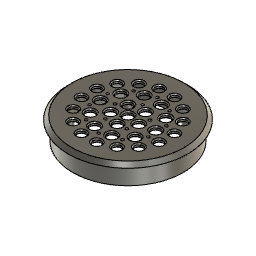
Griglietta aria tonda 60mm v3 (Autodesk Fusion 360 design; units mm, degrees)
Autodesk Fusion 360 part; units mm, degrees
cylinder "PrimitivaCilindro1" add diameter 70 height 2 placed x (1, 0, 0) y (0, 1, 0) z (0, 0, 1) at (0, 0, 0)
sketch "Schizzo2" plane through (0, 0, 2) normal (0, 0, 1) x (-1, 0, 0)
  circle A0 centre (0, 0) radius 35
  circle A1 centre (5, -5) radius 2.4718
  circle A2 centre (6.3004, 3.2102) radius 2.4718
  circle A3 centre (-1.1062, 6.984) radius 2.4718
  circle A4 centre (-6.984, 1.1062) radius 2.4718
  circle A5 centre (-3.2102, -6.3004) radius 2.4718
  circle A6 centre (12.1495, -8.2504) radius 2.5
  circle A7 centre (14.6786, 0.4666) radius 2.5
  circle A8 centre (11.601, 9.0053) radius 2.5
  circle A9 centre (4.0922, 14.1043) radius 2.5
  circle A10 centre (-4.9797, 13.816) radius 2.5
  circle A11 centre (-12.1495, 8.2504) radius 2.5
  circle A12 centre (-14.6786, -0.4666) radius 2.5
  circle A13 centre (-11.601, -9.0053) radius 2.5
  circle A14 centre (-4.0922, -14.1043) radius 2.5
  circle A15 centre (4.9797, -13.816) radius 2.5
  line L0 (16, -16) -> (-16, 16) construction
  circle A16 centre (21.1596, 4.1773) radius 2.2588
  circle A17 centre (17.9503, 11.9568) radius 2.2588
  circle A18 centre (12.0083, 17.9159) radius 2.2588
  circle A19 centre (4.2381, 21.1475) radius 2.2588
  circle A20 centre (-4.1773, 21.1596) radius 2.2588
  circle A21 centre (-11.9568, 17.9503) radius 2.2588
  circle A22 centre (-17.9159, 12.0083) radius 2.2588
  circle A23 centre (-21.1475, 4.2381) radius 2.2588
  circle A24 centre (-21.1596, -4.1773) radius 2.2588
  circle A25 centre (-17.9503, -11.9568) radius 2.2588
  circle A26 centre (-12.0083, -17.9159) radius 2.2588
  circle A27 centre (-4.2381, -21.1475) radius 2.2588
  circle A28 centre (4.1773, -21.1596) radius 2.2588
  circle A29 centre (11.9568, -17.9503) radius 2.2588
  circle A30 centre (17.9159, -12.0083) radius 2.2588
  circle A31 centre (21.1475, -4.2381) radius 2.2588
  dimension "d4" = 360
  dimension "d5" = 5
  dimension "d7" = 360
  constraint coincident L0 A0.centre
  constraint coincident A0.centre origin
  measures "d5" diameter of A6
extrude "Estrusione4" cut sketch "Schizzo2" against normal blind 10 contours A1 | A2 | A3 | A4 | A5 | A6 | A7 | A8 | A9 | A10 | A11 | A12 | A13 | A14 | A15 | A16 | A17 | A18 | A19 | A20 | A21 | A22 | A23 | A24 | A25 | A26 | A27 | A28 | A29 | A30 | A31
sketch "Schizzo3" plane through (0, 0, 0) normal (0, 0, -1) x (1, 0, 0)
  circle A0 centre (0, 0) radius 35
  circle A1 centre (0, 0) radius 30.1
  circle A2 centre (0, 0) radius 29.4
  circle A3 centre (-12.0083, 17.9159) radius 2.2588
  circle A4 centre (3.2102, -6.3004) radius 2.4718
  circle A5 centre (-14.6786, 0.4666) radius 2.5
  circle A6 centre (21.1596, -4.1773) radius 2.2588
  circle A7 centre (21.1475, 4.2381) radius 2.2588
  circle A8 centre (4.9797, 13.816) radius 2.5
  circle A9 centre (11.601, -9.0053) radius 2.5
  circle A10 centre (-21.1475, -4.2381) radius 2.2588
  circle A11 centre (-4.1773, -21.1596) radius 2.2588
  circle A12 centre (14.6786, -0.4666) radius 2.5
  circle A13 centre (-17.9503, 11.9568) radius 2.2588
  circle A14 centre (11.9568, 17.9503) radius 2.2588
  circle A15 centre (1.1062, 6.984) radius 2.4718
  circle A16 centre (-6.3004, 3.2102) radius 2.4718
  circle A17 centre (4.2381, -21.1475) radius 2.2588
  circle A18 centre (4.1773, 21.1596) radius 2.2588
  circle A19 centre (-11.601, 9.0053) radius 2.5
  circle A20 centre (-4.0922, 14.1043) radius 2.5
  circle A21 centre (17.9503, -11.9568) radius 2.2588
  circle A22 centre (17.9159, 12.0083) radius 2.2588
  circle A23 centre (12.1495, 8.2504) radius 2.5
  circle A24 centre (-4.9797, -13.816) radius 2.5
  circle A25 centre (-17.9159, -12.0083) radius 2.2588
  circle A26 centre (-11.9568, -17.9503) radius 2.2588
  circle A27 centre (4.0922, -14.1043) radius 2.5
  circle A28 centre (-21.1596, 4.1773) radius 2.2588
  circle A29 centre (12.0083, -17.9159) radius 2.2588
  circle A30 centre (6.984, 1.1062) radius 2.4718
  circle A31 centre (-5, -5) radius 2.4718
  circle A32 centre (-12.1495, -8.2504) radius 2.5
  circle A33 centre (-4.2381, 21.1475) radius 2.2588
  dimension "d17" = 60.2
  dimension "d18" = 58.8
  constraint concentric A0 A1
  constraint concentric A1 A2
  measures "d17" diameter of A1
  measures "d18" diameter of A2
extrude "Estrusione2" add sketch "Schizzo3" along normal blind 10 contours A1
fillet "Raccordo2" radius 1 1 edges at (-32.6315, -12.6565, 2)
sketch "Schizzo5" plane through (0, 0, 0) normal (0, 0, 1) x (1, 0, 0)
  line L0 (20, 20) -> (-20, 20)
  line L1 (-20, 20) -> (-20, -20)
  line L2 (20, -20) -> (20, 20)
  line L3 (20, 20) -> (-20, -20) construction
  line L4 (-20, 20) -> (20, -20) construction
  line L5 (18.5, 18.5) -> (-18.5, 18.5)
  line L6 (-18.5, 18.5) -> (-18.5, -18.5)
  line L7 (-18.5, -18.5) -> (18.5, -18.5)
  line L8 (18.5, -18.5) -> (18.5, 18.5)
  line L9 (18.5, 18.5) -> (-18.5, -18.5) construction
  line L10 (-18.5, 18.5) -> (18.5, -18.5) construction
  line L11 (16, 16) -> (-16, 16)
  line L12 (-16, 16) -> (-16, -16)
  line L13 (-16, -16) -> (16, -16)
  line L14 (16, -16) -> (16, 16)
  line L15 (16, 16) -> (-16, -16) construction
  line L16 (-16, 16) -> (16, -16) construction
  circle A0 centre (-20, -20) radius 2
  circle A1 centre (-18.5, -18.5) radius 2
  circle A2 centre (-16, -16) radius 2
  circle A3 centre (0, 0) radius 29.4
  circle A4 centre (20, -20) radius 2
  circle A5 centre (20, -20) radius 2
  circle A6 centre (18.5, -18.5) radius 2
  circle A7 centre (16, -16) radius 2
  circle A8 centre (-20, 20) radius 2
  circle A9 centre (-18.5, 18.5) radius 2
  circle A10 centre (-16, 16) radius 2
  circle A11 centre (16, 16) radius 2
  circle A12 centre (18.5, 18.5) radius 2
  circle A13 centre (20, 20) radius 2
  circle A14 centre (-16, 16) radius 0.5
  circle A15 centre (-18.5, 18.5) radius 0.5
  circle A16 centre (-20, 20) radius 0.5
  circle A17 centre (16, 16) radius 0.5
  circle A18 centre (18.5, 18.5) radius 0.5
  circle A19 centre (20, 20) radius 0.5
  circle A20 centre (-20, -20) radius 0.5
  circle A21 centre (-18.5, -18.5) radius 0.5
  circle A22 centre (-16, -16) radius 0.5
  circle A23 centre (16, -16) radius 0.5
  circle A24 centre (18.5, -18.5) radius 0.5
  circle A25 centre (20, -20) radius 0.5
  dimension "d27" = 40
  dimension "d28" = 40
  dimension "d29" = 37
  dimension "d30" = 37
  dimension "d31" = 32
  dimension "d32" = 32
  dimension "d41" = 4
  dimension "d42" = 4
  dimension "d43" = 4
  dimension "d44" = 58.8
  dimension "d45" = 4
  dimension "d46" = 4
  dimension "d47" = 4
  dimension "d48" = 4
  dimension "d49" = 4
  dimension "d50" = 4
  dimension "d51" = 4
  dimension "d52" = 4
  dimension "d53" = 4
  dimension "d54" = 4
  dimension "d55" = 1
  dimension "d56" = 1
  dimension "d57" = 1
  dimension "d58" = 1
  dimension "d59" = 1
  dimension "d60" = 1
  dimension "d61" = 1
  dimension "d62" = 1
  dimension "d63" = 1
  dimension "d64" = 1
  dimension "d65" = 1
  dimension "d66" = 1
  constraint horizontal L0
  constraint perpendicular L0 L1
  constraint parallel L1 L2
  constraint coincident L3 A3.centre
  constraint coincident L4 A3.centre
  constraint coincident A3.centre origin
  constraint horizontal L5
  constraint perpendicular L5 L6
  constraint parallel L5 L7
  constraint parallel L6 L8
  constraint coincident L9 A3.centre
  constraint coincident L10 A3.centre
  constraint horizontal L11
  constraint perpendicular L11 L12
  constraint parallel L11 L13
  constraint parallel L12 L14
  constraint coincident L15 A3.centre
  constraint coincident L16 A3.centre
  constraint coincident L1.end L3.end
  constraint coincident L6.end L7.start
  constraint coincident L12.end L13.start
  constraint coincident L2.start L4.end
  constraint coincident L7.end L8.start
  constraint coincident L13.end L14.start
  constraint coincident L0.end L1.start
  constraint coincident L5.end L6.start
  constraint coincident L11.end L12.start
  constraint coincident L11.start L14.end
  constraint coincident L5.start L8.end
  constraint coincident L0.start L2.end
  constraint concentric A10 A14
  constraint concentric A9 A15
  constraint concentric A8 A16
  constraint concentric A11 A17
  constraint concentric A12 A18
  constraint concentric A13 A19
  constraint concentric A0 A20
  constraint concentric A1 A21
  constraint concentric A2 A22
  constraint concentric A7 A23
  constraint concentric A6 A24
  constraint concentric A5 A25
  measures "d27" distance of L1.end L2.start
  measures "d28" distance of L0.end L1.end
  measures "d29" distance of L6.end L7.end
  measures "d30" distance of L5.end L6.end
  measures "d31" distance of L12.end L13.end
  measures "d32" distance of L11.end L12.end
  measures "d41" diameter of A0
  measures "d42" diameter of A1
  measures "d43" diameter of A2
  measures "d44" diameter of A3
  measures "d45" diameter of A4
  measures "d46" diameter of A5
  measures "d47" diameter of A6
  measures "d48" diameter of A7
  measures "d49" diameter of A8
  measures "d50" diameter of A9
  measures "d51" diameter of A10
  measures "d52" diameter of A11
  measures "d53" diameter of A12
  measures "d54" diameter of A13
  measures "d55" diameter of A14
  measures "d56" diameter of A15
  measures "d57" diameter of A16
  measures "d58" diameter of A17
  measures "d59" diameter of A18
  measures "d60" diameter of A19
  measures "d61" diameter of A20
  measures "d62" diameter of A21
  measures "d63" diameter of A22
  measures "d64" diameter of A23
  measures "d65" diameter of A24
  measures "d66" diameter of A25
extrude "Estrusione5" add sketch "Schizzo5" against normal blind 10 contours L0 L1 A8 A15 A16 | L0 A8 A9 | L0 A8 A9 A16 | L0 L5 A8 A9 A15 | A3 A8 A9 A16 | L1 A8 A9 A16 | L0 A12 A13 | L0 L5 A12 A13 A18 | L5 L6 A9 A10 A15 | L1 L6 A8 A9 A15 | L1 A8 A9 | L0 A12 A13 A19 | L0 L2 A13 A18 A19 | A3 A12 A13 A19 | L5 L8 A11 A12 A18 | L11 L12 A9 A10 A14 | A9 A10 | L11 L14 A11 A12 A17 | A11 A12 | L11 L12 A10 A14 | A0 A1 A3 A20 | L1 L6 A0 A1 A21 | L1 A0 A1 | L2 A12 A13 A19 | L2 L8 A12 A13 A18 | L11 L14 A11 A17 | L2 A12 A13 | L1 A0 A1 A20 | L6 L7 A1 A2 A21 | L1 A0 A1 A20 A21 | L12 L13 A2 A22 | L12 L13 A1 A2 A22 | A3 A4 A5 A6 A25 | L7 A0 A1 A21 | A1 A2 | L2 L8 A4 A5 A6 A24 | L7 L8 A6 A7 A24 | L13 L14 A6 A7 A23 | L13 L14 A7 A23 | L2 A4 A5 A6 A25 | L2 A4 A5 A6 | L7 A4 A5 A6 A24 | L2 A4 A5 A6 A24 A25 | A6 A7
extrude "Estrusione6" add sketch "Schizzo5" against normal blind 5 contours L7 L8 A4 A5 A24 | L7 L8 A24 | L13 L14 A23 | L13 L14 A23 | A4 A5 A24 | L2 A6 A25 | A6 A25 | L2 A6 A25
extrude "Estrusione7" add 3 faces at (-18.3961, -18.32, 0) (-19.8961, -19.82, 0) (-15.9875, -16.1588, 0) along direction (0, 0, -1) blind 5
extrude "Estrusione8" add 3 faces at (-15.8463, 15.9752, 0) (-18.3961, 18.68, 0) (-19.8961, 20.18, 0) along direction (0, 0, -1) blind 5
extrude "Estrusione9" add 3 faces at (16.1368, 15.8392, 0) (18.6039, 18.68, 0) (20.1039, 20.18, 0) along direction (0, 0, -1) blind 5
sketch "Schizzo6" plane through (0, 0, 0) normal (0, 0, -1) x (1, 0, 0)
  circle A0 centre (-12.0083, 17.9159) radius 2.2588
  circle A1 centre (3.2102, -6.3004) radius 2.4718
  circle A2 centre (-14.6786, 0.4666) radius 2.5
  circle A3 centre (21.1596, -4.1773) radius 2.2588
  circle A4 centre (21.1475, 4.2381) radius 2.2588
  circle A5 centre (4.9797, 13.816) radius 2.5
  circle A6 centre (11.601, -9.0053) radius 2.5
  circle A7 centre (-21.1475, -4.2381) radius 2.2588
  circle A8 centre (-4.1773, -21.1596) radius 2.2588
  circle A9 centre (14.6786, -0.4666) radius 2.5
  circle A10 centre (-17.9503, 11.9568) radius 2.2588
  circle A11 centre (11.9568, 17.9503) radius 2.2588
  circle A12 centre (1.1062, 6.984) radius 2.4718
  circle A13 centre (-6.3004, 3.2102) radius 2.4718
  circle A14 centre (4.2381, -21.1475) radius 2.2588
  circle A15 centre (4.1773, 21.1596) radius 2.2588
  circle A16 centre (-11.601, 9.0053) radius 2.5
  circle A17 centre (-4.0922, 14.1043) radius 2.5
  circle A18 centre (17.9503, -11.9568) radius 2.2588
  circle A19 centre (17.9159, 12.0083) radius 2.2588
  circle A20 centre (12.1495, 8.2504) radius 2.5
  circle A21 centre (-4.9797, -13.816) radius 2.5
  circle A22 centre (-17.9159, -12.0083) radius 2.2588
  circle A23 centre (-11.9568, -17.9503) radius 2.2588
  circle A24 centre (4.0922, -14.1043) radius 2.5
  circle A25 centre (-21.1596, 4.1773) radius 2.2588
  circle A26 centre (12.0083, -17.9159) radius 2.2588
  circle A27 centre (6.984, 1.1062) radius 2.4718
  circle A28 centre (-5, -5) radius 2.4718
  circle A29 centre (-12.1495, -8.2504) radius 2.5
  circle A30 centre (-4.2381, 21.1475) radius 2.2588
  arc A31 (20.449, 18.051) -> (21.9506, 19.5584) centre (20, 20) ccw
  arc A32 (17.9114, 16.5886) -> (20.449, 18.051) centre (18.5, 18.5) ccw
  arc A33 (16.5886, 17.9114) -> (17.9114, 16.5886) centre (16, 16) ccw
  arc A34 (18.051, 20.449) -> (16.5886, 17.9114) centre (18.5, 18.5) ccw
  arc A35 (19.5584, 21.9506) -> (18.051, 20.449) centre (20, 20) ccw
  arc A36 (19.5584, 21.9506) -> (-19.5584, 21.9506) centre (0, 0) ccw
  arc A37 (-18.051, 20.449) -> (-19.5584, 21.9506) centre (-20, 20) ccw
  arc A38 (-16.5886, 17.9114) -> (-18.051, 20.449) centre (-18.5, 18.5) ccw
  arc A39 (-17.9114, 16.5886) -> (-16.5886, 17.9114) centre (-16, 16) ccw
  arc A40 (-20.449, 18.051) -> (-17.9114, 16.5886) centre (-18.5, 18.5) ccw
  arc A41 (-21.9506, 19.5584) -> (-20.449, 18.051) centre (-20, 20) ccw
  arc A42 (-21.9506, 19.5584) -> (-21.9506, -19.5584) centre (0, 0) ccw
  arc A43 (-20.449, -18.051) -> (-21.9506, -19.5584) centre (-20, -20) ccw
  arc A44 (-17.9114, -16.5886) -> (-20.449, -18.051) centre (-18.5, -18.5) ccw
  arc A45 (-16.5886, -17.9114) -> (-17.9114, -16.5886) centre (-16, -16) ccw
  arc A46 (-18.051, -20.449) -> (-16.5886, -17.9114) centre (-18.5, -18.5) ccw
  arc A47 (-19.5584, -21.9506) -> (-18.051, -20.449) centre (-20, -20) ccw
  arc A48 (-19.5584, -21.9506) -> (19.5584, -21.9506) centre (0, 0) ccw
  arc A49 (18.051, -20.449) -> (19.5584, -21.9506) centre (20, -20) ccw
  arc A50 (16.5886, -17.9114) -> (18.051, -20.449) centre (18.5, -18.5) ccw
  arc A51 (17.9114, -16.5886) -> (16.5886, -17.9114) centre (16, -16) ccw
  arc A52 (20.449, -18.051) -> (17.9114, -16.5886) centre (18.5, -18.5) ccw
  arc A53 (21.9506, -19.5584) -> (20.449, -18.051) centre (20, -20) ccw
  arc A54 (21.9506, -19.5584) -> (21.9506, 19.5584) centre (0, 0) ccw
  arc A55 (20, -20) -> (20, 20) centre (-17.5, 0) ccw
  arc A56 (-20, -20) -> (20, -20) centre (0, 17.5134) ccw
  arc A57 (-20, 20) -> (-20, -20) centre (21.0472, 0) ccw
  arc A58 (20, 20) -> (-20, 20) centre (0, -17.5) ccw
  arc A59 (20.2824, 20.5294) -> (-20.2824, 20.5294) centre (0, -17.5) ccw
  arc A60 (-20.4538, -20.4375) -> (20.4432, -20.4432) centre (0, 17.5134) ccw
  arc A61 (20.4432, -20.4432) -> (20.4432, 20.4432) centre (-17.5, 0) ccw
  arc A62 (20.4432, 20.4432) -> (-20.4538, 20.4375) centre (0, -17.5) ccw
  arc A63 (-20.4538, 20.4375) -> (-20.4538, -20.4375) centre (21.0472, 0) ccw
  dimension "d77" = 0.6
  dimension "d78" = 0.6
  constraint coincident A49.centre A53.centre
  constraint coincident A31.centre A35.centre
  constraint coincident A43.centre A47.centre
  constraint tangent A40 A57
  constraint coincident A37.centre A41.centre
extrude "Estrusione10" add sketch "Schizzo6" along normal blind 9.4 contours A31 A53 A55 A61 | A35 A37 A58 A59 A62 | A47 A49 A56 A60 | A41 A43 A57 A63
sketch "Schizzo7" plane through (0, 0, 0) normal (0, 0, -1) x (1, 0, 0)
  circle A0 centre (-12.0083, 17.9159) radius 2.2588
  circle A1 centre (3.2102, -6.3004) radius 2.4718
  circle A2 centre (-14.6786, 0.4666) radius 2.5
  circle A3 centre (21.1596, -4.1773) radius 2.2588
  circle A4 centre (21.1475, 4.2381) radius 2.2588
  circle A5 centre (4.9797, 13.816) radius 2.5
  circle A6 centre (11.601, -9.0053) radius 2.5
  circle A7 centre (-21.1475, -4.2381) radius 2.2588
  circle A8 centre (-4.1773, -21.1596) radius 2.2588
  circle A9 centre (14.6786, -0.4666) radius 2.5
  circle A10 centre (-17.9503, 11.9568) radius 2.2588
  circle A11 centre (11.9568, 17.9503) radius 2.2588
  circle A12 centre (1.1062, 6.984) radius 2.4718
  circle A13 centre (-6.3004, 3.2102) radius 2.4718
  circle A14 centre (4.2381, -21.1475) radius 2.2588
  circle A15 centre (4.1773, 21.1596) radius 2.2588
  circle A16 centre (-11.601, 9.0053) radius 2.5
  circle A17 centre (-4.0922, 14.1043) radius 2.5
  circle A18 centre (17.9503, -11.9568) radius 2.2588
  circle A19 centre (17.9159, 12.0083) radius 2.2588
  circle A20 centre (12.1495, 8.2504) radius 2.5
  circle A21 centre (-4.9797, -13.816) radius 2.5
  circle A22 centre (-17.9159, -12.0083) radius 2.2588
  circle A23 centre (-11.9568, -17.9503) radius 2.2588
  circle A24 centre (4.0922, -14.1043) radius 2.5
  circle A25 centre (-21.1596, 4.1773) radius 2.2588
  circle A26 centre (12.0083, -17.9159) radius 2.2588
  circle A27 centre (6.984, 1.1062) radius 2.4718
  circle A28 centre (-5, -5) radius 2.4718
  circle A29 centre (-12.1495, -8.2504) radius 2.5
  circle A30 centre (-4.2381, 21.1475) radius 2.2588
  arc A31 (-20.8364, 18.1833) -> (-20.8364, -18.1833) centre (21.0472, 0) ccw
  arc A32 (-20.449, -18.051) -> (-20.8364, -18.1833) centre (-20, -20) ccw
  arc A33 (-17.9114, -16.5886) -> (-20.449, -18.051) centre (-18.5, -18.5) ccw
  arc A34 (-16.5886, -17.9114) -> (-17.9114, -16.5886) centre (-16, -16) ccw
  arc A35 (-18.051, -20.449) -> (-16.5886, -17.9114) centre (-18.5, -18.5) ccw
  arc A36 (-18.2135, -20.8991) -> (-18.051, -20.449) centre (-20, -20) ccw
  arc A37 (-18.2135, -20.8991) -> (18.2135, -20.8991) centre (0, 17.5134) ccw
  arc A38 (18.051, -20.449) -> (18.2135, -20.8991) centre (20, -20) ccw
  arc A39 (16.5886, -17.9114) -> (18.051, -20.449) centre (18.5, -18.5) ccw
  arc A40 (17.9114, -16.5886) -> (16.5886, -17.9114) centre (16, -16) ccw
  arc A41 (20.449, -18.051) -> (17.9114, -16.5886) centre (18.5, -18.5) ccw
  arc A42 (20.8994, -18.2136) -> (20.449, -18.051) centre (20, -20) ccw
  arc A43 (20.8994, -18.2136) -> (20.8994, 18.2136) centre (-17.5, 0) ccw
  arc A44 (20.449, 18.051) -> (20.8994, 18.2136) centre (20, 20) ccw
  arc A45 (17.9114, 16.5886) -> (20.449, 18.051) centre (18.5, 18.5) ccw
  arc A46 (16.5886, 17.9114) -> (17.9114, 16.5886) centre (16, 16) ccw
  arc A47 (18.051, 20.449) -> (16.5886, 17.9114) centre (18.5, 18.5) ccw
  arc A48 (18.2136, 20.8994) -> (18.051, 20.449) centre (20, 20) ccw
  arc A49 (18.2136, 20.8994) -> (-18.2136, 20.8994) centre (0, -17.5) ccw
  arc A50 (-18.051, 20.449) -> (-18.2136, 20.8994) centre (-20, 20) ccw
  arc A51 (-16.5886, 17.9114) -> (-18.051, 20.449) centre (-18.5, 18.5) ccw
  arc A52 (-17.9114, 16.5886) -> (-16.5886, 17.9114) centre (-16, 16) ccw
  arc A53 (-20.449, 18.051) -> (-17.9114, 16.5886) centre (-18.5, 18.5) ccw
  arc A54 (-20.8364, 18.1833) -> (-20.449, 18.051) centre (-20, 20) ccw
  circle A55 centre (0, 0) radius 2.5
  circle A56 centre (-10, -13) radius 0.75
  circle A57 centre (-0.449, -16.3951) radius 0.75
  circle A58 centre (9.2736, -13.5278) radius 0.75
  circle A59 centre (15.4539, -5.4933) radius 0.75
  circle A60 centre (15.7314, 4.6394) radius 0.75
  circle A61 centre (10, 13) radius 0.75
  circle A62 centre (0.449, 16.3951) radius 0.75
  circle A63 centre (-9.2736, 13.5278) radius 0.75
  circle A64 centre (-15.4539, 5.4933) radius 0.75
  circle A65 centre (-15.7314, -4.6394) radius 0.75
  circle A66 centre (-1, -9) radius 0.75
  circle A67 centre (8.2505, -3.7322) radius 0.75
  circle A68 centre (6.0991, 6.6934) radius 0.75
  circle A69 centre (-4.4811, 7.8689) radius 0.75
  circle A70 centre (-8.8685, -1.8301) radius 0.75
  dimension "d81" = 5
  dimension "d82" = 1.5
  dimension "d84" = 360
  dimension "d85" = 1.5
  dimension "d87" = 360
  constraint coincident A55.centre origin
  measures "d81" diameter of A55
  measures "d82" diameter of A56
  measures "d85" diameter of A66
extrude "Estrusione11" cut sketch "Schizzo7" against normal blind 4 contours A55 | A56 | A57 | A58 | A59 | A60 | A61 | A62 | A63 | A64 | A65 | A66 | A67 | A68 | A69 | A70
sketch "Schizzo8" plane through (0, 0, 0) normal (0, 0, 1) x (1, 0, 0)
  circle A0 centre (0, 0) radius 28.25
  dimension "d90" = 56.5
  constraint coincident A0.centre origin
  measures "d90" diameter of A0
split_face "DividiFaccia1" 4 faces at (26.605, 3.5465, 0) (-26.3601, 3.5319, 0) (3.5465, 26.604, 0) (3.5465, -26.605, 0) by curves path "Schizzo8" along A0
extrude "Estrusione12" add 4 faces at (-23.2271, -16.6422, 0) (-16.5206, 23.3188, 0) (23.3193, -16.52, 0) (-16.52, -23.3193, 0) along direction (0, 0, -1) blind 10
sketch "Schizzo9" plane through (0, 0, 2) normal (0, 0, 1) x (-1, 0, 0)
  circle A0 centre (-10, 13) radius 0.75
  circle A1 centre (15.4539, 5.4933) radius 0.75
  circle A2 centre (-15.4539, -5.4933) radius 0.75
  circle A3 centre (0.449, -16.3951) radius 0.75
  circle A4 centre (1, -9) radius 0.75
  circle A5 centre (8.8685, -1.8301) radius 0.75
  circle A6 centre (4.4811, 7.8689) radius 0.75
  circle A7 centre (9.2736, 13.5278) radius 0.75
  circle A8 centre (-15.7314, 4.6394) radius 0.75
  circle A9 centre (15.7314, -4.6394) radius 0.75
  circle A10 centre (-8.2505, -3.7322) radius 0.75
  circle A11 centre (10, -13) radius 0.75
  circle A12 centre (-9.2736, -13.5278) radius 0.75
  circle A13 centre (0, 0) radius 2.5
  circle A14 centre (-6.0991, 6.6934) radius 0.75
  circle A15 centre (-0.449, 16.3951) radius 0.75
  circle A16 centre (4.2381, 21.1475) radius 2.2588
  circle A17 centre (12.1495, -8.2504) radius 2.5
  circle A18 centre (5, -5) radius 2.4718
  circle A19 centre (-6.984, 1.1062) radius 2.4718
  circle A20 centre (-12.0083, -17.9159) radius 2.2588
  circle A21 centre (21.1596, 4.1773) radius 2.2588
  circle A22 centre (-4.0922, -14.1043) radius 2.5
  circle A23 centre (11.9568, -17.9503) radius 2.2588
  circle A24 centre (17.9159, -12.0083) radius 2.2588
  circle A25 centre (4.9797, -13.816) radius 2.5
  circle A26 centre (-12.1495, 8.2504) radius 2.5
  circle A27 centre (-17.9159, 12.0083) radius 2.2588
  circle A28 centre (-17.9503, -11.9568) radius 2.2588
  circle A29 centre (4.0922, 14.1043) radius 2.5
  circle A30 centre (11.601, 9.0053) radius 2.5
  circle A31 centre (-4.1773, 21.1596) radius 2.2588
  circle A32 centre (-4.2381, -21.1475) radius 2.2588
  circle A33 centre (6.3004, 3.2102) radius 2.4718
  circle A34 centre (-1.1062, 6.984) radius 2.4718
  circle A35 centre (-11.9568, 17.9503) radius 2.2588
  circle A36 centre (17.9503, 11.9568) radius 2.2588
  circle A37 centre (-14.6786, -0.4666) radius 2.5
  circle A38 centre (4.1773, -21.1596) radius 2.2588
  circle A39 centre (21.1475, -4.2381) radius 2.2588
  circle A40 centre (-11.601, -9.0053) radius 2.5
  circle A41 centre (-4.9797, 13.816) radius 2.5
  circle A42 centre (-21.1475, 4.2381) radius 2.2588
  circle A43 centre (-21.1596, -4.1773) radius 2.2588
  circle A44 centre (14.6786, 0.4666) radius 2.5
  circle A45 centre (-3.2102, -6.3004) radius 2.4718
  circle A46 centre (12.0083, 17.9159) radius 2.2588
  circle A47 centre (0, 0) radius 34
  circle A48 centre (0, 0) radius 32.573
  circle A49 centre (0, 0) radius 36
  constraint coincident A13.centre A47.centre
  constraint concentric A48 A49
extrude "Estrusione13" cut sketch "Schizzo9" against normal blind 50 contours A47 | A49
chamfer "Smusso1" distance 2 angle 45 1 edges at (30.3687, 11.7789, 2) measured on face at (0.8316, 26.2338, 2)
chamfer "Smusso2" distance 0.6 angle 45 32 edges at (-2.1322, -21.9643, 2) (-9.9024, -18.7327, 2) (-1.7614, -15.0084, 2) (6.2833, -21.9764, 2) (7.3105, -14.72, 2) (3.4107, -7.8779, 2) (14.0627, -18.7671, 2) (14.4803, -9.1544, 2) (20.0218, -12.8251, 2) (23.2534, -5.0549, 2) (17.0094, -0.4375, 2) (9.2886, -2, 2) (13.9318, 8.1013, 2) (23.2655, 3.3605, 2) (20.0562, 11.14, 2) (14.1142, 17.0991, 2) (6.344, 20.3307, 2) (6.423, 13.2003, 2) (5.5148, 5.4065, 2) (-2.3308, 0.904, 2) (-2.6954, 4.1061, 2) (-2.6489, 12.9119, 2) (-2.0714, 20.3428, 2) (-9.8509, 17.1335, 2) (-9.8186, 7.3463, 2) (-12.3478, -1.3706, 2) (-9.2701, -9.9094, 2) (-3.9958, -4.1041, 2) (-15.8444, -12.7736, 2) (-15.81, 11.1915, 2) (-19.0416, 3.4213, 2) (-19.0537, -4.9941, 2) measured on face at (-9.6121, 23.584, 2) measured on face at (-9.6121, 23.584, 2) measured on face at (-9.6121, 23.584, 2) measured on face at (-9.6121, 23.584, 2) measured on face at (-9.6121, 23.584, 2) measured on face at (-9.6121, 23.584, 2) measured on face at (-9.6121, 23.584, 2) measured on face at (-9.6121, 23.584, 2) measured on face at (-9.6121, 23.584, 2) measured on face at (-9.6121, 23.584, 2) measured on face at (-9.6121, 23.584, 2) measured on face at (-9.6121, 23.584, 2) measured on face at (-9.6121, 23.584, 2) measured on face at (-9.6121, 23.584, 2) measured on face at (-9.6121, 23.584, 2) measured on face at (-9.6121, 23.584, 2) measured on face at (-9.6121, 23.584, 2) measured on face at (-9.6121, 23.584, 2) measured on face at (-9.6121, 23.584, 2) measured on face at (-9.6121, 23.584, 2) measured on face at (-9.6121, 23.584, 2) measured on face at (-9.6121, 23.584, 2) measured on face at (-9.6121, 23.584, 2) measured on face at (-9.6121, 23.584, 2) measured on face at (-9.6121, 23.584, 2) measured on face at (-9.6121, 23.584, 2) measured on face at (-9.6121, 23.584, 2) measured on face at (-9.6121, 23.584, 2) measured on face at (-9.6121, 23.584, 2) measured on face at (-9.6121, 23.584, 2) measured on face at (-9.6121, 23.584, 2) measured on face at (-9.6121, 23.584, 2)
chamfer "Smusso3" distance 0.5 angle 45 32 edges at (-9.2701, -8.1013, 0) (-15.8444, -11.14, 0) (-19.0537, -3.3605, 0) (-19.0416, 5.0549, 0) (-12.3478, 0.4375, 0) (-9.8186, 9.1544, 0) (-15.81, 12.8251, 0) (-9.8509, 18.7671, 0) (-2.0714, 21.9764, 0) (-2.6489, 14.72, 0) (-2.6954, 5.8939, 0) (-3.9958, -2.3163, 0) (-1.7614, -13.2003, 0) (-2.1322, -20.3307, 0) (-9.9024, -17.0991, 0) (6.2833, -20.3428, 0) (3.4107, -6.0902, 0) (7.3105, -12.9119, 0) (14.4803, -7.3463, 0) (14.0627, -17.1335, 0) (9.2886, -0.2123, 0) (5.5148, 7.1942, 0) (-2.3308, -0.904, 0) (6.423, 15.0084, 0) (6.344, 21.9643, 0) (14.1142, 18.7327, 0) (13.9318, 9.9094, 0) (20.0562, 12.7736, 0) (17.0094, 1.3706, 0) (23.2655, 4.9941, 0) (23.2534, -3.4213, 0) (20.0218, -11.1915, 0) measured on face at (-7.4087, 9.2596, 0) measured on face at (-7.4087, 9.2596, 0) measured on face at (-7.4087, 9.2596, 0) measured on face at (-7.4087, 9.2596, 0) measured on face at (-7.4087, 9.2596, 0) measured on face at (-7.4087, 9.2596, 0) measured on face at (-7.4087, 9.2596, 0) measured on face at (-7.4087, 9.2596, 0) measured on face at (-7.4087, 9.2596, 0) measured on face at (-7.4087, 9.2596, 0) measured on face at (-7.4087, 9.2596, 0) measured on face at (-7.4087, 9.2596, 0) measured on face at (-7.4087, 9.2596, 0) measured on face at (-7.4087, 9.2596, 0) measured on face at (-7.4087, 9.2596, 0) measured on face at (-7.4087, 9.2596, 0) measured on face at (-7.4087, 9.2596, 0) measured on face at (-7.4087, 9.2596, 0) measured on face at (-7.4087, 9.2596, 0) measured on face at (-7.4087, 9.2596, 0) measured on face at (-7.4087, 9.2596, 0) measured on face at (-7.4087, 9.2596, 0) measured on face at (-7.4087, 9.2596, 0) measured on face at (-7.4087, 9.2596, 0) measured on face at (-7.4087, 9.2596, 0) measured on face at (-7.4087, 9.2596, 0) measured on face at (-7.4087, 9.2596, 0) measured on face at (-7.4087, 9.2596, 0) measured on face at (-7.4087, 9.2596, 0) measured on face at (-7.4087, 9.2596, 0) measured on face at (-7.4087, 9.2596, 0) measured on face at (-7.4087, 9.2596, 0)
